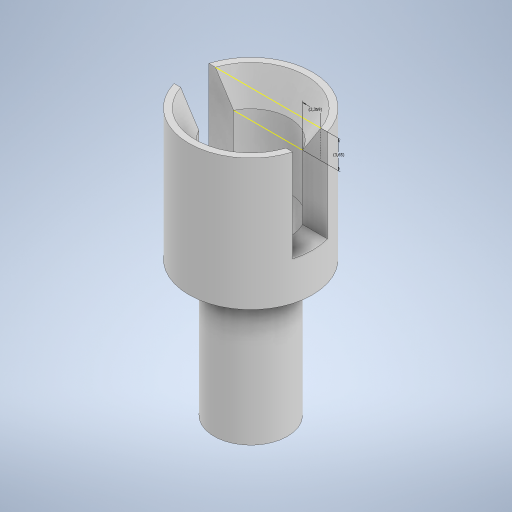
# Autodesk Inventor part: shaft
Saved by Autodesk Inventor 2024 (Build 280153000, 153)
## iProperties
Created: 2025-01-11
Part Number: shaft
Material: Generic
Document SubType Name: Modeling
Designer: kamil
Density: 1 g/cm^3
Appearance: Default
Author: kamil
Autodesk Inventor part; units mm, degrees
ref_plane "YZ Plane" through (0, 0, 0) normal (1, 0, 0) x (0, 1, 0)
ref_plane "XZ Plane" through (0, 0, 0) normal (0, 1, 0) x (-1, 0, 0)
ref_plane "XY Plane" through (0, 0, 0) normal (0, 0, 1) x (1, 0, 0)
sketch "Sketch1" plane through (0, 0, 0) normal (0, 1, 0) x (-1, 0, 0)
  circle A0 centre (0, 0) radius 4.75
  dimension "d0" = 9.5
  constraints: 1 centre point, 1 coincident
  measures "d0" diameter of A0
extrude "Extrusion1" add sketch "Sketch1" along normal blind 17.5
sketch "Sketch2" plane through (0, 17.5, 0) normal (0, 1, 0) x (1, 0, 0)
  circle A0 centre (0, 0) radius 8
  dimension "d3" = 16
  constraints: 1 centre point, 1 coincident
  measures "d3" diameter of A0
extrude "Extrusion2" add sketch "Sketch2" along normal blind 17
sketch "Sketch3" plane through (0, 0, 0) normal (0, 0, 1) x (1, 0, 0)
  line L0 (0, 39.2) -> (0, 22.5)
  line L1 (0, 22.5) -> (10, 39.2)
  line L2 (10, 39.2) -> (0, 39.2)
  line L3 (8, 17.5) -> (-8, 17.5) projected
  line L4 (0, -7.84) -> (0, 47.04) projected
  point P0 (0, 0)
  dimension "d6" = 5
  dimension "d7" = 10
  dimension "d8" = 16.7
  constraints: 6 end point, 1 collinear, 1 perpendicular, 1 vertical
  measures "d6" distance from line of L3 L0.end
  measures "d7" distance of L1.end L0.start
  measures "d8" distance of L0.start L0.end
revolve "Revolution1" cut sketch "Sketch3" angle 360 about axis through (0, -10, 0) along (0, 1, 0)
sketch "Sketch4" plane through (0, 34.5, 0) normal (0, 1, 0) x (1, 0, 0)
  circle A0 centre (0, 0) radius 5
  dimension "d10" = 10
  constraints: 1 centre point, 1 coincident
  measures "d10" diameter of A0
extrude "Extrusion3" cut sketch "Sketch4" against normal blind 12.1
sketch "Sketch5" plane through (0, 34.5, 0) normal (0, 1, 0) x (1, 0, 0)
  line L0 (-8.5, -2.25) -> (8.5, -2.25)
  line L1 (8.5, -2.25) -> (8.5, 2.25)
  line L2 (8.5, 2.25) -> (-8.5, 2.25)
  line L3 (-8.5, 2.25) -> (-8.5, -2.25)
  line L4 (-8.5, -2.25) -> (8.5, 2.25) construction
  line L5 (8.5, -2.25) -> (-8.5, 2.25) construction
  point P0 (0, 0)
  dimension "d13" = 17
  dimension "d14" = 4.5
  constraints: 12 end point, 2 midpoint, 2 parallel, 1 horizontal, 1 perpendicular
  measures "d13" distance of L1.end L2.end
  measures "d14" distance of L0.end L1.end
extrude "Extrusion4" cut sketch "Sketch5" against normal blind 12
sketch "Sketch6" plane through (6.8243, 34.5, -2.25) normal (0, 0, 1) x (1, 0, 0)
  line L0 (-13.6486, 0) -> (0, 0) projected
  line L1 (-11.2894, -3.65) -> (-2.3591, -3.65) projected
  line L2 (0, 0) -> (0, -3.5) construction
  point P0 (-6.8243, -34.5)
  dimension "d17" = 3.65
  dimension "d18" = 2.3591
  constraints: 2 end point, 1 vertical
  measures "d17" distance between parallel lines of L0 L1
  measures "d18" distance from line of L2 L1.end
sketch "Sketch9" plane through (0, 22.4, 0) normal (0, 1, 0) x (1, 0, 0)
  circle A0 centre (0, 0) radius 5 projected
  arc A1 (0, -5) -> (0, 5) centre (0, 0) ccw
  line L0 (0, 0) -> (0, -5) construction
  line L1 (0, 0) -> (0, 5) construction
  line L2 (0, 5) -> (0, -5)
  dimension "d19" = 180
  constraints: 6 end point, 3 point on circle, 1 centre point, 1 coincident
  measures "d19" angle of L0 L1
revolve "Revolution2" cut sketch "Sketch9" angle 360 about axis through (0, 22.4, 0) along (0, 0, -1) picked at (1.0391, 1.3031) contours A0 L2
sketch "Sketch16" plane through (0, 0, 0) normal (0, -1, 0) x (1, 0, 0)
  arc A0 (1.7108, -2.525) -> (-1.7108, -2.525) centre (0, 0) ccw
  line L0 (1.7108, -2.525) -> (-1.7108, -2.525)
  dimension "d55" = 6.1
  dimension "d56" = 0.525
  constraints: 2 end point, 2 point on circle, 1 centre point, 1 coincident, 1 horizontal
  measures "d55" diameter of A0
  measures "d56" distance edge to line of A0 L0
extrude "Extrusion8" cut sketch "Sketch16" against normal blind 12
body "Solid1"
